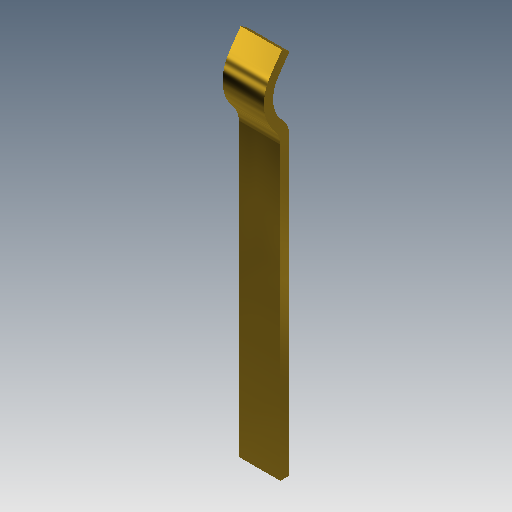
# Autodesk Inventor part: USB Series B Receptacle Terminal
Saved by Autodesk Inventor 2020 (Build 240168000, 168)
## iProperties
Created: 2012-05-08
Material: Bronze, Soft Tin
Document SubType Name: Modeling
Designer: sdarley
Density: 1 g/cm^3
Project: USB Series B Receptacle
Description: USB Series B Receptacle Terminal
Appearance: Gold - Metal
Author: sdarley
Title: USB Series B Receptacle Terminal
Revision Number: 1
Autodesk Inventor part; units mm, degrees
ref_plane "YZ Plane" through (0, 0, 0) normal (1, 0, 0) x (0, 1, 0)
ref_plane "XZ Plane" through (0, 0, 0) normal (0, 1, 0) x (-1, 0, 0)
ref_plane "XY Plane" through (0, 0, 0) normal (0, 0, 1) x (1, 0, 0)
sketch "Sketch1" plane through (0, 0, 0) normal (1, 0, 0) x (0, 1, 0)
  line L0 (-6.5, 0) -> (3.5, 0)
  line L1 (-6.5, 0) -> (-6.5, 0.3)
  line L2 (-6.5, 0.3) -> (3.337, 0.3)
  line L3 (5.5, 0) -> (5.6721, 0.2457)
  line L4 (5.6721, 0.2457) -> (5.1721, 0.5958)
  line L5 (5.5, 0) -> (5, 0.3501)
  arc A0 (5, 0.3501) -> (3.5, 0) centre (4.4069, -0.497) ccw
  arc A1 (5.1721, 0.5958) -> (3.337, 0.3) centre (4.4069, -0.497) ccw
  point P0 (0, 0)
  dimension "d0" = 0.3
  dimension "d3" = 6.5
  dimension "d4" = 10
  dimension "d5" = 35
  dimension "d6" = 2
  dimension "d7" = 0.3
  dimension "d8" = 1.5
  constraints: 12 end point, 4 point on circle, 3 perpendicular, 2 centre point, 2 tangent, 1 concentric, 1 horizontal, 1 horizontal alignment, 1 parallel, 1 point on line
  measures "d0" distance between parallel lines of L0 L2
  measures "d3" distance from line of point (0, 0) L1
  measures "d4" distance from line of L0.end L1
  measures "d5" angle of L0 L5
  measures "d6" distance of L3.start L0.end
  measures "d7" distance between parallel lines of L4 L5
  measures "d8" horizontal distance of L5.end L0.end
extrude "Extrusion1" add sketch "Sketch1" along normal blind 1.35
fillet "Fillet1" radius 0.75 1 edges at (0.675, 3.337, 0.3)
fillet "Fillet2" radius 0.75 1 edges at (0.675, 3.5, 0)
equation "\"d7\" = d0"
body "Solid1"
